Autodesk Fusion 360 part; units mm, degrees
(part 9 of 10)
  line L2725 (-28.0448, 8.6201) -> (-28.0163, 8.6133)
  line L2726 (-19.682, 10.0004) -> (-19.6496, 9.968)
  line L2727 (-19.6496, 9.968) -> (-19.645, 9.945)
  line L2728 (-19.645, 9.945) -> (-19.645, -4.025)
  line L2729 (-19.645, -4.025) -> (-19.6496, -4.048)
  line L2730 (-19.6496, -4.048) -> (-19.682, -4.0804)
  line L2731 (-19.682, -4.0804) -> (-19.705, -4.085)
  line L2732 (-19.705, -4.085) -> (-33.675, -4.085)
  line L2733 (-33.675, -4.085) -> (-33.698, -4.0804)
  line L2734 (-33.698, -4.0804) -> (-33.7304, -4.048)
  line L2735 (-33.7304, -4.048) -> (-33.735, -4.025)
  line L2736 (-33.735, -4.025) -> (-33.735, 9.945)
  line L2737 (-33.735, 9.945) -> (-33.7304, 9.968)
  line L2738 (-33.7304, 9.968) -> (-33.698, 10.0004)
  line L2739 (-33.698, 10.0004) -> (-33.675, 10.005)
  line L2740 (-33.675, 10.005) -> (-19.705, 10.005)
  line L2741 (-19.705, 10.005) -> (-19.682, 10.0004)
  line L2742 (-33.615, 9.885) -> (-33.615, -3.965)
  line L2743 (-33.615, -3.965) -> (-19.765, -3.965)
  line L2744 (-19.765, -3.965) -> (-19.765, 9.885)
  line L2745 (-19.765, 9.885) -> (-33.615, 9.885)
  line L2746 (27.428, 16.5404) -> (27.4604, 16.508)
  line L2747 (27.4604, 16.508) -> (27.465, 16.485)
  line L2748 (27.465, 16.485) -> (27.465, 2.515)
  line L2749 (27.465, 2.515) -> (27.4604, 2.492)
  line L2750 (27.4604, 2.492) -> (27.428, 2.4596)
  line L2751 (27.428, 2.4596) -> (27.405, 2.455)
  line L2752 (27.405, 2.455) -> (13.435, 2.455)
  line L2753 (13.435, 2.455) -> (13.412, 2.4596)
  line L2754 (13.412, 2.4596) -> (13.3796, 2.492)
  line L2755 (13.3796, 2.492) -> (13.375, 2.515)
  line L2756 (13.375, 2.515) -> (13.375, 16.485)
  line L2757 (13.375, 16.485) -> (13.3796, 16.508)
  line L2758 (13.3796, 16.508) -> (13.412, 16.5404)
  line L2759 (13.412, 16.5404) -> (13.435, 16.545)
  line L2760 (13.435, 16.545) -> (27.405, 16.545)
  line L2761 (27.405, 16.545) -> (27.428, 16.5404)
  line L2762 (13.495, 16.425) -> (13.495, 2.575)
  line L2763 (13.495, 2.575) -> (27.345, 2.575)
  line L2764 (27.345, 2.575) -> (27.345, 16.425)
  line L2765 (27.345, 16.425) -> (13.495, 16.425)
  line L2766 (-19.682, 25.0904) -> (-19.6496, 25.058)
  line L2767 (-19.6496, 25.058) -> (-19.645, 25.035)
  line L2768 (-19.645, 25.035) -> (-19.645, 11.065)
  line L2769 (-19.645, 11.065) -> (-19.6496, 11.042)
  line L2770 (-19.6496, 11.042) -> (-19.682, 11.0096)
  line L2771 (-19.682, 11.0096) -> (-19.705, 11.005)
  line L2772 (-19.705, 11.005) -> (-33.675, 11.005)
  line L2773 (-33.675, 11.005) -> (-33.698, 11.0096)
  line L2774 (-33.698, 11.0096) -> (-33.7304, 11.042)
  line L2775 (-33.7304, 11.042) -> (-33.735, 11.065)
  line L2776 (-33.735, 11.065) -> (-33.735, 25.035)
  line L2777 (-33.735, 25.035) -> (-33.7304, 25.058)
  line L2778 (-33.7304, 25.058) -> (-33.698, 25.0904)
  line L2779 (-33.698, 25.0904) -> (-33.675, 25.095)
  line L2780 (-33.675, 25.095) -> (-19.705, 25.095)
  line L2781 (-19.705, 25.095) -> (-19.682, 25.0904)
  line L2782 (-33.615, 24.975) -> (-33.615, 11.125)
  line L2783 (-33.615, 11.125) -> (-19.765, 11.125)
  line L2784 (-19.765, 11.125) -> (-19.765, 24.975)
  line L2785 (-19.765, 24.975) -> (-33.615, 24.975)
  line L2786 (19.0465, 17.9935) -> (19.0484, 17.9936)
  line L2787 (19.0484, 17.9936) -> (19.051, 17.993)
  line L2788 (19.051, 17.993) -> (19.0537, 17.9927)
  line L2789 (19.0537, 17.9927) -> (19.0555, 17.992)
  line L2790 (19.0555, 17.992) -> (19.0628, 17.9903)
  line L2791 (19.0628, 17.9903) -> (19.2056, 17.9427)
  line L2792 (19.2056, 17.9427) -> (19.219, 17.9367)
  line L2793 (19.219, 17.9367) -> (19.2412, 17.9175)
  line L2794 (19.2412, 17.9175) -> (19.2542, 17.8914)
  line L2795 (19.2542, 17.8914) -> (19.2563, 17.8622)
  line L2796 (19.2563, 17.8622) -> (19.2471, 17.8344)
  line L2797 (19.2471, 17.8344) -> (19.2279, 17.8123)
  line L2798 (19.2279, 17.8123) -> (19.2017, 17.7992)
  line L2799 (19.2017, 17.7992) -> (19.1725, 17.7972)
  line L2800 (19.1725, 17.7972) -> (19.1582, 17.8004)
  line L2801 (19.1582, 17.8004) -> (19.0269, 17.8442)
  line L2802 (19.0269, 17.8442) -> (18.8187, 17.8442)
  line L2803 (18.8187, 17.8442) -> (18.7501, 17.8099)
  line L2804 (18.7501, 17.8099) -> (18.7197, 17.7795)
  line L2805 (18.7197, 17.7795) -> (18.6855, 17.711)
  line L2806 (18.6855, 17.711) -> (18.6855, 17.6512)
  line L2807 (18.6855, 17.6512) -> (18.7197, 17.5827)
  line L2808 (18.7197, 17.5827) -> (18.7501, 17.5522)
  line L2809 (18.7501, 17.5522) -> (18.8271, 17.5138)
  line L2810 (18.8271, 17.5138) -> (19.0096, 17.4681)
  line L2811 (19.0096, 17.4681) -> (19.0107, 17.4677)
  line L2812 (19.0107, 17.4677) -> (19.0112, 17.4677)
  line L2813 (19.0112, 17.4677) -> (19.0173, 17.4654)
  line L2814 (19.0173, 17.4654) -> (19.0235, 17.4632)
  line L2815 (19.0235, 17.4632) -> (19.0239, 17.4629)
  line L2816 (19.0239, 17.4629) -> (19.025, 17.4625)
  line L2817 (19.025, 17.4625) -> (19.1202, 17.4148)
  line L2818 (19.1202, 17.4148) -> (19.1265, 17.4109)
  line L2819 (19.1265, 17.4109) -> (19.1283, 17.4101)
  line L2820 (19.1283, 17.4101) -> (19.1304, 17.4084)
  line L2821 (19.1304, 17.4084) -> (19.1327, 17.407)
  line L2822 (19.1327, 17.407) -> (19.1339, 17.4055)
  line L2823 (19.1339, 17.4055) -> (19.1397, 17.4008)
  line L2824 (19.1397, 17.4008) -> (19.1873, 17.3532)
  line L2825 (19.1873, 17.3532) -> (19.192, 17.3474)
  line L2826 (19.192, 17.3474) -> (19.1935, 17.3461)
  line L2827 (19.1935, 17.3461) -> (19.195, 17.3439)
  line L2828 (19.195, 17.3439) -> (19.1966, 17.3418)
  line L2829 (19.1966, 17.3418) -> (19.1974, 17.34)
  line L2830 (19.1974, 17.34) -> (19.2014, 17.3337)
  line L2831 (19.2014, 17.3337) -> (19.249, 17.2384)
  line L2832 (19.249, 17.2384) -> (19.2542, 17.2247)
  line L2833 (19.2542, 17.2247) -> (19.2544, 17.222)
  line L2834 (19.2544, 17.222) -> (19.2555, 17.2195)
  line L2835 (19.2555, 17.2195) -> (19.2569, 17.2049)
  line L2836 (19.2569, 17.2049) -> (19.2569, 17.1097)
  line L2837 (19.2569, 17.1097) -> (19.2555, 17.095)
  line L2838 (19.2555, 17.095) -> (19.2544, 17.0925)
  line L2839 (19.2544, 17.0925) -> (19.2542, 17.0898)
  line L2840 (19.2542, 17.0898) -> (19.249, 17.0761)
  line L2841 (19.249, 17.0761) -> (19.2014, 16.9809)
  line L2842 (19.2014, 16.9809) -> (19.1974, 16.9746)
  line L2843 (19.1974, 16.9746) -> (19.1966, 16.9728)
  line L2844 (19.1966, 16.9728) -> (19.195, 16.9707)
  line L2845 (19.195, 16.9707) -> (19.1935, 16.9684)
  line L2846 (19.1935, 16.9684) -> (19.192, 16.9671)
  line L2847 (19.192, 16.9671) -> (19.1873, 16.9614)
  line L2848 (19.1873, 16.9614) -> (19.1397, 16.9138)
  line L2849 (19.1397, 16.9138) -> (19.134, 16.909)
  line L2850 (19.134, 16.909) -> (19.1327, 16.9075)
  line L2851 (19.1327, 16.9075) -> (19.1304, 16.9061)
  line L2852 (19.1304, 16.9061) -> (19.1283, 16.9044)
  line L2853 (19.1283, 16.9044) -> (19.1265, 16.9037)
  line L2854 (19.1265, 16.9037) -> (19.1202, 16.8997)
  line L2855 (19.1202, 16.8997) -> (19.025, 16.8521)
  line L2856 (19.025, 16.8521) -> (19.0112, 16.8468)
  line L2857 (19.0112, 16.8468) -> (19.0085, 16.8467)
  line L2858 (19.0085, 16.8467) -> (19.0061, 16.8456)
  line L2859 (19.0061, 16.8456) -> (18.9914, 16.8442)
  line L2860 (18.9914, 16.8442) -> (18.7533, 16.8442)
  line L2861 (18.7533, 16.8442) -> (18.7459, 16.8449)
  line L2862 (18.7459, 16.8449) -> (18.744, 16.8448)
  line L2863 (18.744, 16.8448) -> (18.7414, 16.8454)
  line L2864 (18.7414, 16.8454) -> (18.7387, 16.8456)
  line L2865 (18.7387, 16.8456) -> (18.7369, 16.8464)
  line L2866 (18.7369, 16.8464) -> (18.7296, 16.848)
  line L2867 (18.7296, 16.848) -> (18.5868, 16.8956)
  line L2868 (18.5868, 16.8956) -> (18.5733, 16.9016)
  line L2869 (18.5733, 16.9016) -> (18.5512, 16.9208)
  line L2870 (18.5512, 16.9208) -> (18.5381, 16.947)
  line L2871 (18.5381, 16.947) -> (18.5361, 16.9762)
  line L2872 (18.5361, 16.9762) -> (18.5453, 17.0039)
  line L2873 (18.5453, 17.0039) -> (18.5645, 17.0261)
  line L2874 (18.5645, 17.0261) -> (18.5907, 17.0391)
  line L2875 (18.5907, 17.0391) -> (18.6199, 17.0412)
  line L2876 (18.6199, 17.0412) -> (18.6342, 17.038)
  line L2877 (18.6342, 17.038) -> (18.7655, 16.9942)
  line L2878 (18.7655, 16.9942) -> (18.9737, 16.9942)
  line L2879 (18.9737, 16.9942) -> (19.0422, 17.0284)
  line L2880 (19.0422, 17.0284) -> (19.0726, 17.0588)
  line L2881 (19.0726, 17.0588) -> (19.1069, 17.1274)
  line L2882 (19.1069, 17.1274) -> (19.1069, 17.1872)
  line L2883 (19.1069, 17.1872) -> (19.0726, 17.2557)
  line L2884 (19.0726, 17.2557) -> (19.0422, 17.2861)
  line L2885 (19.0422, 17.2861) -> (18.9653, 17.3246)
  line L2886 (18.9653, 17.3246) -> (18.7828, 17.3702)
  line L2887 (18.7828, 17.3702) -> (18.7817, 17.3706)
  line L2888 (18.7817, 17.3706) -> (18.7811, 17.3707)
  line L2889 (18.7811, 17.3707) -> (18.7751, 17.373)
  line L2890 (18.7751, 17.373) -> (18.7689, 17.3752)
  line L2891 (18.7689, 17.3752) -> (18.7685, 17.3755)
  line L2892 (18.7685, 17.3755) -> (18.7674, 17.3759)
  line L2893 (18.7674, 17.3759) -> (18.6722, 17.4235)
  line L2894 (18.6722, 17.4235) -> (18.6659, 17.4275)
  line L2895 (18.6659, 17.4275) -> (18.664, 17.4282)
  line L2896 (18.664, 17.4282) -> (18.662, 17.4299)
  line L2897 (18.662, 17.4299) -> (18.6597, 17.4314)
  line L2898 (18.6597, 17.4314) -> (18.6584, 17.4329)
  line L2899 (18.6584, 17.4329) -> (18.6527, 17.4376)
  line L2900 (18.6527, 17.4376) -> (18.6051, 17.4852)
  line L2901 (18.6051, 17.4852) -> (18.6003, 17.4909)
  line L2902 (18.6003, 17.4909) -> (18.5988, 17.4922)
  line L2903 (18.5988, 17.4922) -> (18.5974, 17.4945)
  line L2904 (18.5974, 17.4945) -> (18.5957, 17.4966)
  line L2905 (18.5957, 17.4966) -> (18.595, 17.4984)
  line L2906 (18.595, 17.4984) -> (18.591, 17.5047)
  line L2907 (18.591, 17.5047) -> (18.5434, 17.5999)
  line L2908 (18.5434, 17.5999) -> (18.5381, 17.6137)
  line L2909 (18.5381, 17.6137) -> (18.5379, 17.6163)
  line L2910 (18.5379, 17.6163) -> (18.5369, 17.6188)
  line L2911 (18.5369, 17.6188) -> (18.5355, 17.6335)
  line L2912 (18.5355, 17.6335) -> (18.5355, 17.7287)
  line L2913 (18.5355, 17.7287) -> (18.5369, 17.7433)
  line L2914 (18.5369, 17.7433) -> (18.5379, 17.7458)
  line L2915 (18.5379, 17.7458) -> (18.5381, 17.7485)
  line L2916 (18.5381, 17.7485) -> (18.5434, 17.7622)
  line L2917 (18.5434, 17.7622) -> (18.591, 17.8575)
  line L2918 (18.591, 17.8575) -> (18.595, 17.8638)
  line L2919 (18.595, 17.8638) -> (18.5957, 17.8656)
  line L2920 (18.5957, 17.8656) -> (18.5974, 17.8677)
  line L2921 (18.5974, 17.8677) -> (18.5988, 17.8699)
  line L2922 (18.5988, 17.8699) -> (18.6003, 17.8712)
  line L2923 (18.6003, 17.8712) -> (18.6051, 17.877)
  line L2924 (18.6051, 17.877) -> (18.6527, 17.9246)
  line L2925 (18.6527, 17.9246) -> (18.6584, 17.9293)
  line L2926 (18.6584, 17.9293) -> (18.6597, 17.9308)
  line L2927 (18.6597, 17.9308) -> (18.662, 17.9322)
  line L2928 (18.662, 17.9322) -> (18.664, 17.9339)
  line L2929 (18.664, 17.9339) -> (18.6659, 17.9347)
  line L2930 (18.6659, 17.9347) -> (18.6722, 17.9386)
  line L2931 (18.6722, 17.9386) -> (18.7674, 17.9863)
  line L2932 (18.7674, 17.9863) -> (18.7811, 17.9915)
  line L2933 (18.7811, 17.9915) -> (18.7838, 17.9917)
  line L2934 (18.7838, 17.9917) -> (18.7863, 17.9927)
  line L2935 (18.7863, 17.9927) -> (18.801, 17.9942)
  line L2936 (18.801, 17.9942) -> (19.039, 17.9942)
  line L2937 (19.039, 17.9942) -> (19.0465, 17.9935)
  line L2938 (20.9986, 17.9927) -> (21.0061, 17.9927)
  line L2939 (21.0061, 17.9927) -> (21.0128, 17.9899)
  line L2940 (21.0128, 17.9899) -> (21.0201, 17.9885)
  line L2941 (21.0201, 17.9885) -> (21.0262, 17.9844)
  line L2942 (21.0262, 17.9844) -> (21.0331, 17.9815)
  line L2943 (21.0331, 17.9815) -> (21.0383, 17.9763)
  line L2944 (21.0383, 17.9763) -> (21.0444, 17.9723)
  line L2945 (21.0444, 17.9723) -> (21.0485, 17.9661)
  line L2946 (21.0485, 17.9661) -> (21.0538, 17.9608)
  line L2947 (21.0538, 17.9608) -> (21.0566, 17.9541)
  line L2948 (21.0566, 17.9541) -> (21.0607, 17.948)
  line L2949 (21.0607, 17.948) -> (21.0621, 17.9407)
  line L2950 (21.0621, 17.9407) -> (21.065, 17.9338)
  line L2951 (21.065, 17.9338) -> (21.0664, 17.9193)
  line L2952 (26.0664, 17.9193) -> (26.0664, 17.9193)
  line L2953 (26.0664, 17.9193) -> (26.0664, 17.9192)
  line L2954 (26.0664, 17.9192) -> (26.0664, 17.9192)
  line L2955 (21.0664, 17.9192) -> (21.0664, 16.9942)
  line L2956 (21.0664, 16.9942) -> (21.2771, 16.9942)
  line L2957 (21.2771, 16.9942) -> (21.2918, 16.9927)
  line L2958 (21.2918, 16.9927) -> (21.3188, 16.9815)
  line L2959 (21.3188, 16.9815) -> (21.3395, 16.9608)
  line L2960 (21.3395, 16.9608) -> (21.3507, 16.9338)
  line L2961 (21.3507, 16.9338) -> (21.3507, 16.9045)
  line L2962 (21.3507, 16.9045) -> (21.3395, 16.8775)
  line L2963 (21.3395, 16.8775) -> (21.3188, 16.8568)
  line L2964 (21.3188, 16.8568) -> (21.2918, 16.8456)
  line L2965 (21.2918, 16.8456) -> (21.2771, 16.8442)
  line L2966 (21.2771, 16.8442) -> (20.7057, 16.8442)
  line L2967 (20.7057, 16.8442) -> (20.6911, 16.8456)
  line L2968 (20.6911, 16.8456) -> (20.664, 16.8568)
  line L2969 (20.664, 16.8568) -> (20.6434, 16.8775)
  line L2970 (20.6434, 16.8775) -> (20.6322, 16.9045)
  line L2971 (20.6322, 16.9045) -> (20.6322, 16.9338)
  line L2972 (20.6322, 16.9338) -> (20.6434, 16.9608)
  line L2973 (20.6434, 16.9608) -> (20.664, 16.9815)
  line L2974 (20.664, 16.9815) -> (20.6911, 16.9927)
  line L2975 (20.6911, 16.9927) -> (20.7057, 16.9942)
  line L2976 (20.7057, 16.9942) -> (20.9164, 16.9942)
  line L2977 (20.9164, 16.9942) -> (20.9164, 17.6905)
  line L2978 (20.9164, 17.6905) -> (20.854, 17.6281)
  line L2979 (20.854, 17.6281) -> (20.8482, 17.6233)
  line L2980 (20.8482, 17.6233) -> (20.8469, 17.6218)
  line L2981 (20.8469, 17.6218) -> (20.8447, 17.6204)
  line L2982 (20.8447, 17.6204) -> (20.8426, 17.6187)
  line L2983 (20.8426, 17.6187) -> (20.8408, 17.618)
  line L2984 (20.8408, 17.618) -> (20.8345, 17.614)
  line L2985 (20.8345, 17.614) -> (20.7393, 17.5664)
  line L2986 (20.7393, 17.5664) -> (20.7255, 17.5611)
  line L2987 (20.7255, 17.5611) -> (20.6963, 17.5591)
  line L2988 (20.6963, 17.5591) -> (20.6686, 17.5683)
  line L2989 (20.6686, 17.5683) -> (20.6465, 17.5875)
  line L2990 (20.6465, 17.5875) -> (20.6334, 17.6137)
  line L2991 (20.6334, 17.6137) -> (20.6313, 17.6428)
  line L2992 (20.6313, 17.6428) -> (20.6406, 17.6706)
  line L2993 (20.6406, 17.6706) -> (20.6597, 17.6927)
  line L2994 (20.6597, 17.6927) -> (20.6722, 17.7005)
  line L2995 (20.6722, 17.7005) -> (20.7565, 17.7427)
  line L2996 (20.7565, 17.7427) -> (20.8379, 17.8241)
  line L2997 (20.8379, 17.8241) -> (20.929, 17.9608)
  line L2998 (25.929, 17.9608) -> (25.9291, 17.9608)
  line L2999 (25.9291, 17.9608) -> (25.9291, 17.9608)
  line L3000 (25.9291, 17.9608) -> (25.9291, 17.9609)
  line L3001 (20.9291, 17.9609) -> (20.9383, 17.9722)
  line L3002 (20.9383, 17.9722) -> (20.9445, 17.9763)
  line L3003 (20.9445, 17.9763) -> (20.9498, 17.9815)
  line L3004 (20.9498, 17.9815) -> (20.9565, 17.9844)
  line L3005 (20.9565, 17.9844) -> (20.9627, 17.9884)
  line L3006 (20.9627, 17.9884) -> (20.9699, 17.9899)
  line L3007 (20.9699, 17.9899) -> (20.9768, 17.9927)
  line L3008 (20.9768, 17.9927) -> (20.9841, 17.9927)
  line L3009 (20.9841, 17.9927) -> (20.9913, 17.9942)
  line L3010 (20.9913, 17.9942) -> (20.9986, 17.9927)
  line L3011 (22.0061, 17.9927) -> (22.0085, 17.9917)
  line L3012 (22.0085, 17.9917) -> (22.0112, 17.9915)
  line L3013 (22.0112, 17.9915) -> (22.025, 17.9863)
  line L3014 (22.025, 17.9863) -> (22.1202, 17.9386)
  line L3015 (22.1202, 17.9386) -> (22.1265, 17.9347)
  line L3016 (22.1265, 17.9347) -> (22.1283, 17.9339)
  line L3017 (22.1283, 17.9339) -> (22.1304, 17.9322)
  line L3018 (22.1304, 17.9322) -> (22.1327, 17.9308)
  line L3019 (22.1327, 17.9308) -> (22.1339, 17.9293)
  line L3020 (22.1339, 17.9293) -> (22.1397, 17.9246)
  line L3021 (22.1397, 17.9246) -> (22.1873, 17.877)
  line L3022 (22.1873, 17.877) -> (22.192, 17.8712)
  line L3023 (22.192, 17.8712) -> (22.1935, 17.8699)
  line L3024 (22.1935, 17.8699) -> (22.195, 17.8677)
  line L3025 (22.195, 17.8677) -> (22.1966, 17.8656)
  line L3026 (22.1966, 17.8656) -> (22.1974, 17.8638)
  line L3027 (22.1974, 17.8638) -> (22.2014, 17.8575)
  line L3028 (22.2014, 17.8575) -> (22.249, 17.7622)
  line L3029 (22.249, 17.7622) -> (22.2494, 17.7612)
  line L3030 (22.2494, 17.7612) -> (22.2497, 17.7607)
  line L3031 (22.2497, 17.7607) -> (22.2519, 17.7546)
  line L3032 (22.2519, 17.7546) -> (22.2542, 17.7485)
  line L3033 (22.2542, 17.7485) -> (22.2543, 17.748)
  line L3034 (22.2543, 17.748) -> (22.2547, 17.7469)
  line L3035 (22.2547, 17.7469) -> (22.3023, 17.5564)
  line L3036 (22.3023, 17.5564) -> (22.3027, 17.5539)
  line L3037 (22.3027, 17.5539) -> (22.3031, 17.5529)
  line L3038 (22.3031, 17.5529) -> (22.3036, 17.5473)
  line L3039 (22.3036, 17.5473) -> (22.3044, 17.5419)
  line L3040 (22.3044, 17.5419) -> (22.3043, 17.5408)
  line L3041 (22.3043, 17.5408) -> (22.3045, 17.5382)
  line L3042 (22.3045, 17.5382) -> (22.3045, 17.3001)
  line L3043 (22.3045, 17.3001) -> (22.3043, 17.2976)
  line L3044 (22.3043, 17.2976) -> (22.3044, 17.2965)
  line L3045 (22.3044, 17.2965) -> (22.3036, 17.291)
  line L3046 (22.3036, 17.291) -> (22.3031, 17.2855)
  line L3047 (22.3031, 17.2855) -> (22.3027, 17.2845)
  line L3048 (22.3027, 17.2845) -> (22.3023, 17.2819)
  line L3049 (22.3023, 17.2819) -> (22.2547, 17.0915)
  line L3050 (22.2547, 17.0915) -> (22.2543, 17.0904)
  line L3051 (22.2543, 17.0904) -> (22.2542, 17.0898)
  line L3052 (22.2542, 17.0898) -> (22.2519, 17.0838)
  line L3053 (22.2519, 17.0838) -> (22.2497, 17.0776)
  line L3054 (22.2497, 17.0776) -> (22.2494, 17.0772)
  line L3055 (22.2494, 17.0772) -> (22.249, 17.0761)
  line L3056 (22.249, 17.0761) -> (22.2014, 16.9809)
  line L3057 (22.2014, 16.9809) -> (22.1974, 16.9746)
  line L3058 (22.1974, 16.9746) -> (22.1966, 16.9728)
  line L3059 (22.1966, 16.9728) -> (22.195, 16.9707)
  line L3060 (22.195, 16.9707) -> (22.1935, 16.9684)
  line L3061 (22.1935, 16.9684) -> (22.192, 16.9671)
  line L3062 (22.192, 16.9671) -> (22.1873, 16.9614)
  line L3063 (22.1873, 16.9614) -> (22.1397, 16.9138)
  line L3064 (22.1397, 16.9138) -> (22.134, 16.909)
  line L3065 (22.134, 16.909) -> (22.1327, 16.9075)
  line L3066 (22.1327, 16.9075) -> (22.1304, 16.9061)
  line L3067 (22.1304, 16.9061) -> (22.1283, 16.9044)
  line L3068 (22.1283, 16.9044) -> (22.1265, 16.9037)
  line L3069 (22.1265, 16.9037) -> (22.1202, 16.8997)
  line L3070 (22.1202, 16.8997) -> (22.025, 16.8521)
  line L3071 (22.025, 16.8521) -> (22.0112, 16.8468)
  line L3072 (22.0112, 16.8468) -> (22.0085, 16.8467)
  line L3073 (22.0085, 16.8467) -> (22.0061, 16.8456)
  line L3074 (22.0061, 16.8456) -> (21.9914, 16.8442)
  line L3075 (21.9914, 16.8442) -> (21.8962, 16.8442)
  line L3076 (21.8962, 16.8442) -> (21.8816, 16.8456)
  line L3077 (21.8816, 16.8456) -> (21.8791, 16.8467)
  line L3078 (21.8791, 16.8467) -> (21.8764, 16.8468)
  line L3079 (21.8764, 16.8468) -> (21.8626, 16.8521)
  line L3080 (21.8626, 16.8521) -> (21.7674, 16.8997)
  line L3081 (21.7674, 16.8997) -> (21.7611, 16.9037)
  line L3082 (21.7611, 16.9037) -> (21.7593, 16.9044)
  line L3083 (21.7593, 16.9044) -> (21.7572, 16.9061)
  line L3084 (21.7572, 16.9061) -> (21.755, 16.9075)
  line L3085 (21.755, 16.9075) -> (21.7537, 16.909)
  line L3086 (21.7537, 16.909) -> (21.7479, 16.9138)
  line L3087 (21.7479, 16.9138) -> (21.7003, 16.9614)
  line L3088 (21.7003, 16.9614) -> (21.6956, 16.9671)
  line L3089 (21.6956, 16.9671) -> (21.6941, 16.9684)
  line L3090 (21.6941, 16.9684) -> (21.6927, 16.9707)
  line L3091 (21.6927, 16.9707) -> (21.691, 16.9728)
  line L3092 (21.691, 16.9728) -> (21.6902, 16.9746)
  line L3093 (21.6902, 16.9746) -> (21.6863, 16.9809)
  line L3094 (21.6863, 16.9809) -> (21.6386, 17.0761)
  line L3095 (21.6386, 17.0761) -> (21.6382, 17.0772)
  line L3096 (21.6382, 17.0772) -> (21.6379, 17.0776)
  line L3097 (21.6379, 17.0776) -> (21.6357, 17.0838)
  line L3098 (21.6357, 17.0838) -> (21.6334, 17.0898)
  line L3099 (21.6334, 17.0898) -> (21.6333, 17.0904)
  line L3100 (21.6333, 17.0904) -> (21.633, 17.0915)
  line L3101 (21.633, 17.0915) -> (21.5853, 17.2819)
  line L3102 (21.5853, 17.2819) -> (21.585, 17.2845)
  line L3103 (21.585, 17.2845) -> (21.5845, 17.2855)
  line L3104 (21.5845, 17.2855) -> (21.584, 17.291)
  line L3105 (21.584, 17.291) -> (21.5832, 17.2965)
  line L3106 (21.5832, 17.2965) -> (21.5833, 17.2976)
  line L3107 (21.5833, 17.2976) -> (21.5831, 17.3001)
  line L3108 (21.5831, 17.3001) -> (21.5831, 17.5382)
  line L3109 (21.5831, 17.5382) -> (21.5833, 17.5408)
  line L3110 (21.5833, 17.5408) -> (21.5832, 17.5419)
  line L3111 (21.5832, 17.5419) -> (21.584, 17.5473)
  line L3112 (21.584, 17.5473) -> (21.5845, 17.5529)
  line L3113 (21.5845, 17.5529) -> (21.585, 17.5539)
  line L3114 (21.585, 17.5539) -> (21.5853, 17.5564)
  line L3115 (21.5853, 17.5564) -> (21.633, 17.7469)
  line L3116 (21.633, 17.7469) -> (21.6333, 17.748)
  line L3117 (21.6333, 17.748) -> (21.6334, 17.7485)
  line L3118 (21.6334, 17.7485) -> (21.6357, 17.7546)
  line L3119 (21.6357, 17.7546) -> (21.6379, 17.7607)
  line L3120 (21.6379, 17.7607) -> (21.6382, 17.7612)
  line L3121 (21.6382, 17.7612) -> (21.6386, 17.7622)
  line L3122 (21.6386, 17.7622) -> (21.6863, 17.8575)
  line L3123 (21.6863, 17.8575) -> (21.6902, 17.8638)
  line L3124 (21.6902, 17.8638) -> (21.691, 17.8656)
  line L3125 (21.691, 17.8656) -> (21.6927, 17.8677)
  line L3126 (21.6927, 17.8677) -> (21.6941, 17.8699)
  line L3127 (21.6941, 17.8699) -> (21.6956, 17.8712)
  line L3128 (21.6956, 17.8712) -> (21.7003, 17.877)
  line L3129 (21.7003, 17.877) -> (21.7479, 17.9246)
  line L3130 (21.7479, 17.9246) -> (21.7537, 17.9293)
  line L3131 (21.7537, 17.9293) -> (21.755, 17.9308)
  line L3132 (21.755, 17.9308) -> (21.7572, 17.9322)
  line L3133 (21.7572, 17.9322) -> (21.7593, 17.9339)
  line L3134 (21.7593, 17.9339) -> (21.7611, 17.9347)
  line L3135 (21.7611, 17.9347) -> (21.7674, 17.9386)
  line L3136 (21.7674, 17.9386) -> (21.8626, 17.9863)
  line L3137 (21.8626, 17.9863) -> (21.8764, 17.9915)
  line L3138 (21.8764, 17.9915) -> (21.8791, 17.9917)
  line L3139 (21.8791, 17.9917) -> (21.8816, 17.9927)
  line L3140 (21.8816, 17.9927) -> (21.8962, 17.9942)
  line L3141 (21.8962, 17.9942) -> (21.9914, 17.9942)
  line L3142 (21.9914, 17.9942) -> (22.0061, 17.9927)
  line L3143 (21.8454, 17.8099) -> (21.815, 17.7795)
  line L3144 (21.815, 17.7795) -> (21.7765, 17.7025)
  line L3145 (21.7765, 17.7025) -> (21.7331, 17.529)
  line L3146 (21.7331, 17.529) -> (21.7331, 17.3094)
  line L3147 (21.7331, 17.3094) -> (21.7765, 17.1358)
  line L3148 (21.7765, 17.1358) -> (21.815, 17.0588)
  line L3149 (21.815, 17.0588) -> (21.8454, 17.0284)
  line L3150 (21.8454, 17.0284) -> (21.9139, 16.9942)
  line L3151 (21.9139, 16.9942) -> (21.9737, 16.9942)
  line L3152 (21.9737, 16.9942) -> (22.0422, 17.0284)
  line L3153 (22.0422, 17.0284) -> (22.0726, 17.0588)
  line L3154 (22.0726, 17.0588) -> (22.1111, 17.1358)
  line L3155 (22.1111, 17.1358) -> (22.1545, 17.3094)
  line L3156 (22.1545, 17.3094) -> (22.1545, 17.529)
  line L3157 (22.1545, 17.529) -> (22.1111, 17.7025)
  line L3158 (22.1111, 17.7025) -> (22.0726, 17.7795)
  line L3159 (22.0726, 17.7795) -> (22.0422, 17.8099)
  line L3160 (22.0422, 17.8099) -> (21.9737, 17.8442)
  line L3161 (21.9737, 17.8442) -> (21.9139, 17.8442)
  line L3162 (21.9139, 17.8442) -> (21.8454, 17.8099)
  line L3163 (20.4037, 17.9874) -> (20.4274, 17.9702)
  line L3164 (20.4274, 17.9702) -> (20.4427, 17.9453)
  line L3165 (20.4427, 17.9453) -> (20.4473, 17.9164)
  line L3166 (20.4473, 17.9164) -> (20.4453, 17.9018)
  line L3167 (20.4453, 17.9018) -> (20.2072, 16.9018)
  line L3168 (20.2072, 16.9018) -> (20.2055, 16.8968)
  line L3169 (20.2055, 16.8968) -> (20.2053, 16.895)
  line L3170 (20.2053, 16.895) -> (20.2043, 16.8934)
  line L3171 (20.2043, 16.8934) -> (20.2025, 16.8879)
  line L3172 (20.2025, 16.8879) -> (20.1961, 16.8791)
  line L3173 (20.1961, 16.8791) -> (20.1906, 16.8697)
  line L3174 (20.1906, 16.8697) -> (20.1876, 16.8673)
  line L3175 (20.1876, 16.8673) -> (20.1853, 16.8642)
  line L3176 (20.1853, 16.8642) -> (20.176, 16.8585)
  line L3177 (20.176, 16.8585) -> (20.1674, 16.8519)
  line L3178 (20.1674, 16.8519) -> (20.1637, 16.8509)
  line L3179 (20.1637, 16.8509) -> (20.1604, 16.8489)
  line L3180 (20.1604, 16.8489) -> (20.1496, 16.8471)
  line L3181 (20.1496, 16.8471) -> (20.1391, 16.8443)
  line L3182 (20.1391, 16.8443) -> (20.1353, 16.8448)
  line L3183 (20.1353, 16.8448) -> (20.1315, 16.8442)
  line L3184 (20.1315, 16.8442) -> (20.1209, 16.8468)
  line L3185 (20.1209, 16.8468) -> (20.1101, 16.8482)
  line L3186 (20.1101, 16.8482) -> (20.1068, 16.8501)
  line L3187 (20.1068, 16.8501) -> (20.103, 16.851)
  line L3188 (20.103, 16.851) -> (20.0942, 16.8574)
  line L3189 (20.0942, 16.8574) -> (20.0848, 16.8629)
  line L3190 (20.0848, 16.8629) -> (20.0824, 16.8659)
  line L3191 (20.0824, 16.8659) -> (20.0793, 16.8682)
  line L3192 (20.0793, 16.8682) -> (20.0736, 16.8774)
  line L3193 (20.0736, 16.8774) -> (20.067, 16.8861)
  line L3194 (20.067, 16.8861) -> (20.065, 16.8915)
  line L3195 (20.065, 16.8915) -> (20.064, 16.8931)
  line L3196 (20.064, 16.8931) -> (20.0637, 16.8949)
  line L3197 (20.0637, 16.8949) -> (20.0618, 16.8999)
  line L3198 (20.0618, 16.8999) -> (19.9438, 17.3424)
  line L3199 (19.9438, 17.3424) -> (19.8258, 16.8999)
  line L3200 (19.8258, 16.8999) -> (19.8239, 16.8949)
  line L3201 (19.8239, 16.8949) -> (19.8236, 16.8931)
  line L3202 (19.8236, 16.8931) -> (19.8227, 16.8915)
  line L3203 (19.8227, 16.8915) -> (19.8206, 16.8861)
  line L3204 (19.8206, 16.8861) -> (19.814, 16.8774)
  line L3205 (19.814, 16.8774) -> (19.8083, 16.8682)
  line L3206 (19.8083, 16.8682) -> (19.8052, 16.8659)
  line L3207 (19.8052, 16.8659) -> (19.8029, 16.8629)
  line L3208 (19.8029, 16.8629) -> (19.7934, 16.8574)
  line L3209 (19.7934, 16.8574) -> (19.7846, 16.851)
  line L3210 (19.7846, 16.851) -> (19.7809, 16.8501)
  line L3211 (19.7809, 16.8501) -> (19.7775, 16.8482)
  line L3212 (19.7775, 16.8482) -> (19.7667, 16.8468)
  line L3213 (19.7667, 16.8468) -> (19.7561, 16.8442)
  line L3214 (19.7561, 16.8442) -> (19.7523, 16.8448)
  line L3215 (19.7523, 16.8448) -> (19.7485, 16.8443)
  line L3216 (19.7485, 16.8443) -> (19.738, 16.8471)
  line L3217 (19.738, 16.8471) -> (19.7272, 16.8489)
  line L3218 (19.7272, 16.8489) -> (19.724, 16.8509)
  line L3219 (19.724, 16.8509) -> (19.7202, 16.8519)
  line L3220 (19.7202, 16.8519) -> (19.7116, 16.8585)
  line L3221 (19.7116, 16.8585) -> (19.7023, 16.8642)
  line L3222 (19.7023, 16.8642) -> (19.7001, 16.8673)
  line L3223 (19.7001, 16.8673) -> (19.697, 16.8697)
  line L3224 (19.697, 16.8697) -> (19.6915, 16.8791)
  line L3225 (19.6915, 16.8791) -> (19.6852, 16.8879)
  line L3226 (19.6852, 16.8879) -> (19.6833, 16.8934)
  line L3227 (19.6833, 16.8934) -> (19.6823, 16.895)
  line L3228 (19.6823, 16.895) -> (19.6821, 16.8968)
  line L3229 (19.6821, 16.8968) -> (19.6804, 16.9018)
  line L3230 (19.6804, 16.9018) -> (19.4423, 17.9018)
  line L3231 (19.4423, 17.9018) -> (19.4403, 17.9164)
  line L3232 (19.4403, 17.9164) -> (19.4449, 17.9453)
  line L3233 (19.4449, 17.9453) -> (19.4603, 17.9702)
  line L3234 (19.4603, 17.9702) -> (19.484, 17.9874)
  line L3235 (19.484, 17.9874) -> (19.5124, 17.9941)
  line L3236 (19.5124, 17.9941) -> (19.5413, 17.9895)
  line L3237 (19.5413, 17.9895) -> (19.5663, 17.9742)
  line L3238 (19.5663, 17.9742) -> (19.5834, 17.9505)
  line L3239 (19.5834, 17.9505) -> (19.5882, 17.9366)
  line L3240 (19.5882, 17.9366) -> (19.7574, 17.2257)
  line L3241 (19.7574, 17.2257) -> (19.8713, 17.6528)
  line L3242 (19.8713, 17.6528) -> (19.8726, 17.6562)
  line L3243 (19.8726, 17.6562) -> (19.8728, 17.6577)
  line L3244 (19.8728, 17.6577) -> (19.8738, 17.6594)
  line L3245 (19.8738, 17.6594) -> (19.8765, 17.6666)
  line L3246 (19.8765, 17.6666) -> (19.8825, 17.6744)
  line L3247 (19.8825, 17.6744) -> (19.8875, 17.683)
  line L3248 (19.8875, 17.683) -> (19.8913, 17.6859)
  line L3249 (19.8913, 17.6859) -> (19.8943, 17.6898)
  line L3250 (19.8943, 17.6898) -> (19.9029, 17.6948)
  line L3251 (19.9029, 17.6948) -> (19.9107, 17.7008)
  line L3252 (19.9107, 17.7008) -> (19.9154, 17.702)
  line L3253 (19.9154, 17.702) -> (19.9196, 17.7045)
  line L3254 (19.9196, 17.7045) -> (19.9294, 17.7058)
  line L3255 (19.9294, 17.7058) -> (19.939, 17.7083)
  line L3256 (19.939, 17.7083) -> (19.9438, 17.7077)
  line L3257 (19.9438, 17.7077) -> (19.9486, 17.7083)
  line L3258 (19.9486, 17.7083) -> (19.9582, 17.7058)
  line L3259 (19.9582, 17.7058) -> (19.968, 17.7045)
  line L3260 (19.968, 17.7045) -> (19.9722, 17.702)
  line L3261 (19.9722, 17.702) -> (19.9769, 17.7008)
  line L3262 (19.9769, 17.7008) -> (19.9848, 17.6948)
  line L3263 (19.9848, 17.6948) -> (19.9933, 17.6898)
  line L3264 (19.9933, 17.6898) -> (19.9963, 17.6859)
  line L3265 (19.9963, 17.6859) -> (20.0001, 17.683)
  line L3266 (20.0001, 17.683) -> (20.0051, 17.6744)
  line L3267 (20.0051, 17.6744) -> (20.0111, 17.6666)
  line L3268 (20.0111, 17.6666) -> (20.0138, 17.6594)
  line L3269 (20.0138, 17.6594) -> (20.0148, 17.6577)
  line L3270 (20.0148, 17.6577) -> (20.015, 17.6562)
  line L3271 (20.015, 17.6562) -> (20.0163, 17.6528)
  line L3272 (20.0163, 17.6528) -> (20.1302, 17.2257)
  line L3273 (20.1302, 17.2257) -> (20.2994, 17.9366)
  line L3274 (20.2994, 17.9366) -> (20.3042, 17.9505)
  line L3275 (20.3042, 17.9505) -> (20.3214, 17.9742)
  line L3276 (20.3214, 17.9742) -> (20.3463, 17.9895)
  line L3277 (20.3463, 17.9895) -> (20.3752, 17.9941)
  line L3278 (20.3752, 17.9941) -> (20.4037, 17.9874)
  line L3279 (-0.5862, 50.7707) -> (-0.5518, 50.7363)
  line L3280 (-0.5518, 50.7363) -> (-0.547, 50.712)
  line L3281 (-0.547, 50.712) -> (-0.547, 49.3506)
  line L3282 (-0.547, 49.3506) -> (1.7895, 49.3506)
  line L3283 (1.7895, 49.3506) -> (1.8115, 49.3462)
  line L3284 (1.8115, 49.3462) -> (2.0576, 49.3251)
  line L3285 (2.0576, 49.3251) -> (2.3192, 49.2686)
  line L3286 (2.3192, 49.2686) -> (2.5716, 49.1793)
  line L3287 (2.5716, 49.1793) -> (2.8107, 49.0587)
  line L3288 (2.8107, 49.0587) -> (3.0325, 48.9088)
  line L3289 (3.0325, 48.9088) -> (3.2334, 48.7319)
  line L3290 (3.2334, 48.7319) -> (3.4103, 48.5309)
  line L3291 (3.4103, 48.5309) -> (3.5603, 48.3092)
  line L3292 (3.5603, 48.3092) -> (3.6808, 48.0701)
  line L3293 (3.6808, 48.0701) -> (3.7701, 47.8177)
  line L3294 (3.7701, 47.8177) -> (3.8266, 47.556)
  line L3295 (3.8266, 47.556) -> (3.8475, 47.313)
  line L3296 (3.8475, 47.313) -> (3.8482, 47.3123)
  line L3297 (3.8482, 47.3123) -> (3.853, 47.288)
  line L3298 (3.853, 47.288) -> (3.853, 30.288)
  line L3299 (3.853, 30.288) -> (3.8482, 30.2637)
  line L3300 (3.8482, 30.2637) -> (3.8479, 30.2634)
  line L3301 (3.8479, 30.2634) -> (3.8319, 30.0191)
  line L3302 (3.8319, 30.0191) -> (3.7793, 29.7548)
  line L3303 (3.7793, 29.7548) -> (3.6927, 29.4997)
  line L3304 (3.6927, 29.4997) -> (3.5735, 29.258)
  line L3305 (3.5735, 29.258) -> (3.4238, 29.0339)
  line L3306 (3.4238, 29.0339) -> (3.2461, 28.8313)
  line L3307 (3.2461, 28.8313) -> (3.0435, 28.6537)
  line L3308 (3.0435, 28.6537) -> (2.8195, 28.504)
  line L3309 (2.8195, 28.504) -> (2.5778, 28.3848)
  line L3310 (2.5778, 28.3848) -> (2.3227, 28.2982)
  line L3311 (2.3227, 28.2982) -> (2.0584, 28.2456)
  line L3312 (2.0584, 28.2456) -> (1.8141, 28.2296)
  line L3313 (1.8141, 28.2296) -> (1.8138, 28.2293)
  line L3314 (1.8138, 28.2293) -> (1.7895, 28.2245)
  line L3315 (1.7895, 28.2245) -> (-12.0105, 28.2245)
  line L3316 (-12.0105, 28.2245) -> (-12.0348, 28.2293)
  line L3317 (-12.0348, 28.2293) -> (-12.0355, 28.23)
  line L3318 (-12.0355, 28.23) -> (-12.2785, 28.2509)
  line L3319 (-12.2785, 28.2509) -> (-12.5402, 28.3074)
  line L3320 (-12.5402, 28.3074) -> (-12.7926, 28.3967)
  line L3321 (-12.7926, 28.3967) -> (-13.0316, 28.5173)
  line L3322 (-13.0316, 28.5173) -> (-13.2534, 28.6673)
  line L3323 (-13.2534, 28.6673) -> (-13.4543, 28.8441)
  line L3324 (-13.4543, 28.8441) -> (-13.6312, 29.0451)
  line L3325 (-13.6312, 29.0451) -> (-13.7812, 29.2669)
  line L3326 (-13.7812, 29.2669) -> (-13.9018, 29.5059)
  line L3327 (-13.9018, 29.5059) -> (-13.9911, 29.7583)
  line L3328 (-13.9911, 29.7583) -> (-14.0476, 30.0199)
  line L3329 (-14.0476, 30.0199) -> (-14.0685, 30.263)
  line L3330 (-14.0685, 30.263) -> (-14.0692, 30.2637)
  line L3331 (-14.0692, 30.2637) -> (-14.074, 30.288)
  line L3332 (-14.074, 30.288) -> (-14.074, 47.288)
  line L3333 (-14.074, 47.288) -> (-14.0692, 47.3123)
  line L3334 (-14.0692, 47.3123) -> (-14.0685, 47.313)
  line L3335 (-14.0685, 47.313) -> (-14.0476, 47.556)
  line L3336 (-14.0476, 47.556) -> (-13.9911, 47.8177)
  line L3337 (-13.9911, 47.8177) -> (-13.9018, 48.0701)
  line L3338 (-13.9018, 48.0701) -> (-13.7813, 48.3092)
  line L3339 (-13.7813, 48.3092) -> (-13.6313, 48.5309)
  line L3340 (-13.6313, 48.5309) -> (-13.4544, 48.7319)
  line L3341 (-13.4544, 48.7319) -> (-13.2535, 48.9088)
  line L3342 (-13.2535, 48.9088) -> (-13.0317, 49.0587)
  line L3343 (-13.0317, 49.0587) -> (-12.7926, 49.1793)
  line L3344 (-12.7926, 49.1793) -> (-12.5402, 49.2686)
  line L3345 (-12.5402, 49.2686) -> (-12.2786, 49.3251)
  line L3346 (-12.2786, 49.3251) -> (-12.0325, 49.3462)
  line L3347 (-12.0325, 49.3462) -> (-12.0105, 49.3506)
  line L3348 (-12.0105, 49.3506) -> (-9.674, 49.3506)
  line L3349 (-9.674, 49.3506) -> (-9.674, 50.712)
  line L3350 (-9.674, 50.712) -> (-9.6692, 50.7363)
  line L3351 (-9.6692, 50.7363) -> (-9.6348, 50.7707)
  line L3352 (-9.6348, 50.7707) -> (-9.6105, 50.7755)
  line L3353 (-9.6105, 50.7755) -> (-0.6105, 50.7755)
  line L3354 (-0.6105, 50.7755) -> (-0.5862, 50.7707)
  line L3355 (1.7895, 49.2236) -> (-0.547, 49.2236)
  line L3356 (-0.547, 49.2236) -> (-0.547, 43.3587)
  line L3357 (-0.547, 43.3587) -> (-0.5518, 43.3344)
  line L3358 (-0.5518, 43.3344) -> (-0.5862, 43.3)
  line L3359 (-0.5862, 43.3) -> (-0.6105, 43.2952)
  line L3360 (-0.6105, 43.2952) -> (-9.6105, 43.2952)
  line L3361 (-9.6105, 43.2952) -> (-9.6348, 43.3)
  line L3362 (-9.6348, 43.3) -> (-9.6692, 43.3344)
  line L3363 (-9.6692, 43.3344) -> (-9.674, 43.3587)
  line L3364 (-9.674, 43.3587) -> (-9.674, 49.2236)
  line L3365 (-9.674, 49.2236) -> (-12.0105, 49.2236)
  line L3366 (-12.0105, 49.2236) -> (-12.0305, 49.2275)
  line L3367 (-12.0305, 49.2275) -> (-12.1357, 49.2253)
  line L3368 (-12.1357, 49.2253) -> (-12.3858, 49.1877)
  line L3369 (-12.3858, 49.1877) -> (-12.6292, 49.1187)
  line L3370 (-12.6292, 49.1187) -> (-12.8619, 49.0193)
  line L3371 (-12.8619, 49.0193) -> (-13.08, 48.8913)
  line L3372 (-13.08, 48.8913) -> (-13.2802, 48.7365)
  line L3373 (-13.2802, 48.7365) -> (-13.4591, 48.5577)
  line L3374 (-13.4591, 48.5577) -> (-13.6138, 48.3575)
  line L3375 (-13.6138, 48.3575) -> (-13.7419, 48.1393)
  line L3376 (-13.7419, 48.1393) -> (-13.8412, 47.9067)
  line L3377 (-13.8412, 47.9067) -> (-13.9102, 47.6633)
  line L3378 (-13.9102, 47.6633) -> (-13.9478, 47.4131)
  line L3379 (-13.9478, 47.4131) -> (-13.9501, 47.3038)
  line L3380 (-13.9501, 47.3038) -> (-13.947, 47.288)
  line L3381 (-13.947, 47.288) -> (-13.947, 30.288)
  line L3382 (-13.947, 30.288) -> (-13.9501, 30.2722)
  line L3383 (-13.9501, 30.2722) -> (-13.9478, 30.1628)
  line L3384 (-13.9478, 30.1628) -> (-13.9102, 29.9127)
  line L3385 (-13.9102, 29.9127) -> (-13.8412, 29.6693)
  line L3386 (-13.8412, 29.6693) -> (-13.7418, 29.4367)
  line L3387 (-13.7418, 29.4367) -> (-13.6137, 29.2185)
  line L3388 (-13.6137, 29.2185) -> (-13.459, 29.0184)
  line L3389 (-13.459, 29.0184) -> (-13.2801, 28.8395)
  line L3390 (-13.2801, 28.8395) -> (-13.08, 28.6848)
  line L3391 (-13.08, 28.6848) -> (-12.8618, 28.5567)
  line L3392 (-12.8618, 28.5567) -> (-12.6292, 28.4573)
  line L3393 (-12.6292, 28.4573) -> (-12.3858, 28.3883)
  line L3394 (-12.3858, 28.3883) -> (-12.1356, 28.3507)
  line L3395 (-12.1356, 28.3507) -> (-12.0263, 28.3483)
  line L3396 (-12.0263, 28.3483) -> (-12.0105, 28.3515)
  line L3397 (-12.0105, 28.3515) -> (1.7895, 28.3515)
  line L3398 (1.7895, 28.3515) -> (1.8071, 28.348)
  line L3399 (1.8071, 28.348) -> (1.9167, 28.348)
  line L3400 (1.9167, 28.348) -> (2.1688, 28.3812)
  line L3401 (2.1688, 28.3812) -> (2.4144, 28.447)
  line L3402 (2.4144, 28.447) -> (2.6494, 28.5443)
  line L3403 (2.6494, 28.5443) -> (2.8696, 28.6715)
  line L3404 (2.8696, 28.6715) -> (3.0714, 28.8263)
  line L3405 (3.0714, 28.8263) -> (3.2512, 29.0061)
  line L3406 (3.2512, 29.0061) -> (3.406, 29.2079)
  line L3407 (3.406, 29.2079) -> (3.5332, 29.4281)
  line L3408 (3.5332, 29.4281) -> (3.6305, 29.6631)
  line L3409 (3.6305, 29.6631) -> (3.6963, 29.9087)
  line L3410 (3.6963, 29.9087) -> (3.7295, 30.1608)
  line L3411 (3.7295, 30.1608) -> (3.7295, 30.2704)
  line L3412 (3.7295, 30.2704) -> (3.726, 30.288)
  line L3413 (3.726, 30.288) -> (3.726, 47.288)
  line L3414 (3.726, 47.288) -> (3.7291, 47.3038)
  line L3415 (3.7291, 47.3038) -> (3.7268, 47.4131)
  line L3416 (3.7268, 47.4131) -> (3.6892, 47.6633)
  line L3417 (3.6892, 47.6633) -> (3.6202, 47.9067)
  line L3418 (3.6202, 47.9067) -> (3.5209, 48.1393)
  line L3419 (3.5209, 48.1393) -> (3.3928, 48.3575)
  line L3420 (3.3928, 48.3575) -> (3.2381, 48.5577)
  line L3421 (3.2381, 48.5577) -> (3.0592, 48.7365)
  line L3422 (3.0592, 48.7365) -> (2.859, 48.8913)
  line L3423 (2.859, 48.8913) -> (2.6409, 49.0193)
  line L3424 (2.6409, 49.0193) -> (2.4082, 49.1187)
  line L3425 (2.4082, 49.1187) -> (2.1648, 49.1877)
  line L3426 (2.1648, 49.1877) -> (1.9147, 49.2253)
  line L3427 (1.9147, 49.2253) -> (1.8095, 49.2275)
  line L3428 (1.8095, 49.2275) -> (1.7895, 49.2236)
  line L3429 (-9.547, 49.2236) -> (-9.547, 43.4222)
  line L3430 (-9.547, 43.4222) -> (-0.674, 43.4222)
  line L3431 (-0.674, 43.4222) -> (-0.674, 49.2236)
  line L3432 (-0.674, 49.2236) -> (-9.547, 49.2236)
  line L3433 (-9.547, 50.6485) -> (-9.547, 49.3506)
  line L3434 (-9.547, 49.3506) -> (-0.674, 49.3506)
  line L3435 (-0.674, 49.3506) -> (-0.674, 50.6485)
  line L3436 (-0.674, 50.6485) -> (-9.547, 50.6485)
  line L3437 (-33.1806, 36.5339) -> (-33.1461, 36.4994)
  line L3438 (-33.1461, 36.4994) -> (-33.1274, 36.4544)
  line L3439 (-33.1274, 36.4544) -> (-33.125, 36.43)
  line L3440 (-33.125, 36.43) -> (-33.125, 32.725)
  line L3441 (-33.125, 32.725) -> (-21.575, 32.725)
  line L3442 (-21.575, 32.725) -> (-21.575, 36.43)
  line L3443 (-21.575, 36.43) -> (-21.5726, 36.4544)
  line L3444 (-21.5726, 36.4544) -> (-21.5539, 36.4994)
  line L3445 (-21.5539, 36.4994) -> (-21.5194, 36.5339)
  line L3446 (-21.5194, 36.5339) -> (-21.4744, 36.5526)
  line L3447 (-21.4744, 36.5526) -> (-21.4256, 36.5526)
  line L3448 (-21.4256, 36.5526) -> (-21.3806, 36.5339)
  line L3449 (-21.3806, 36.5339) -> (-21.3461, 36.4994)
  line L3450 (-21.3461, 36.4994) -> (-21.3274, 36.4544)
  line L3451 (-21.3274, 36.4544) -> (-21.325, 36.43)
  line L3452 (-21.325, 36.43) -> (-21.325, 32.6)
  line L3453 (-21.325, 32.6) -> (-21.3274, 32.5756)
  line L3454 (-21.3274, 32.5756) -> (-21.3461, 32.5306)
  line L3455 (-21.3461, 32.5306) -> (-21.3806, 32.4961)
  line L3456 (-21.3806, 32.4961) -> (-21.4256, 32.4774)
  line L3457 (-21.4256, 32.4774) -> (-21.45, 32.475)
  line L3458 (-21.45, 32.475) -> (-33.25, 32.475)
  line L3459 (-33.25, 32.475) -> (-33.2744, 32.4774)
  line L3460 (-33.2744, 32.4774) -> (-33.3194, 32.4961)
  line L3461 (-33.3194, 32.4961) -> (-33.3539, 32.5306)
  line L3462 (-33.3539, 32.5306) -> (-33.3726, 32.5756)
  line L3463 (-33.3726, 32.5756) -> (-33.375, 32.6)
  line L3464 (-33.375, 32.6) -> (-33.375, 36.43)
  line L3465 (-33.375, 36.43) -> (-33.3726, 36.4544)
  line L3466 (-33.3726, 36.4544) -> (-33.3539, 36.4994)
  line L3467 (-33.3539, 36.4994) -> (-33.3194, 36.5339)
  line L3468 (-33.3194, 36.5339) -> (-33.2744, 36.5526)
  line L3469 (-33.2744, 36.5526) -> (-33.2256, 36.5526)
  line L3470 (-33.2256, 36.5526) -> (-33.1806, 36.5339)
  line L3471 (-26.8182, 41.7301) -> (-26.471, 41.6509)
  line L3472 (-26.471, 41.6509) -> (-26.135, 41.5333)
  line L3473 (-26.135, 41.5333) -> (-25.8142, 41.3788)
  line L3474 (-25.8142, 41.3788) -> (-25.5127, 41.1894)
  line L3475 (-25.5127, 41.1894) -> (-25.2343, 40.9674)
  line L3476 (-25.2343, 40.9674) -> (-24.9826, 40.7156)
  line L3477 (-24.9826, 40.7156) -> (-24.7606, 40.4373)
  line L3478 (-24.7606, 40.4373) -> (-24.5712, 40.1358)
  line L3479 (-24.5712, 40.1358) -> (-24.4167, 39.815)
  line L3480 (-24.4167, 39.815) -> (-24.2991, 39.479)
  line L3481 (-24.2991, 39.479) -> (-24.2199, 39.1318)
  line L3482 (-24.2199, 39.1318) -> (-24.18, 38.778)
  line L3483 (-24.18, 38.778) -> (-24.18, 38.422)
  line L3484 (-24.18, 38.422) -> (-24.2199, 38.0682)
  line L3485 (-24.2199, 38.0682) -> (-24.2991, 37.721)
  line L3486 (-24.2991, 37.721) -> (-24.4167, 37.385)
  line L3487 (-24.4167, 37.385) -> (-24.5712, 37.0642)
  line L3488 (-24.5712, 37.0642) -> (-24.7606, 36.7627)
  line L3489 (-24.7606, 36.7627) -> (-24.9826, 36.4844)
  line L3490 (-24.9826, 36.4843) -> (-25.2343, 36.2326)
  line L3491 (-25.2343, 36.2326) -> (-25.5127, 36.0106)
  line L3492 (-25.5127, 36.0106) -> (-25.8142, 35.8212)
  line L3493 (-25.8142, 35.8212) -> (-26.135, 35.6667)
  line L3494 (-26.135, 35.6667) -> (-26.471, 35.5491)
  line L3495 (-26.471, 35.5491) -> (-26.8182, 35.4699)
  line L3496 (-26.8182, 35.4699) -> (-27.172, 35.43)
  line L3497 (-27.172, 35.43) -> (-27.528, 35.43)
  line L3498 (-27.528, 35.43) -> (-27.8818, 35.4699)
  line L3499 (-27.8818, 35.4699) -> (-28.229, 35.5491)
  line L3500 (-28.229, 35.5491) -> (-28.565, 35.6667)
  line L3501 (-28.565, 35.6667) -> (-28.8858, 35.8212)
  line L3502 (-28.8858, 35.8212) -> (-29.1873, 36.0106)
  line L3503 (-29.1873, 36.0106) -> (-29.4656, 36.2326)
  line L3504 (-29.4656, 36.2326) -> (-29.7174, 36.4843)
  line L3505 (-29.7174, 36.4843) -> (-29.9394, 36.7627)
  line L3506 (-29.9394, 36.7627) -> (-30.1288, 37.0642)
  line L3507 (-30.1288, 37.0642) -> (-30.2833, 37.385)
  line L3508 (-30.2833, 37.385) -> (-30.4009, 37.721)
  line L3509 (-30.4009, 37.721) -> (-30.4801, 38.0682)
  line L3510 (-30.4801, 38.0682) -> (-30.52, 38.422)
  line L3511 (-30.52, 38.422) -> (-30.52, 38.7643)
  line L3512 (-30.52, 38.7643) -> (-30.52, 38.778)
  line L3513 (-30.52, 38.778) -> (-30.4801, 39.1318)
  line L3514 (-30.4801, 39.1318) -> (-30.4009, 39.479)
  line L3515 (-30.4009, 39.479) -> (-30.2833, 39.815)
  line L3516 (-30.2833, 39.815) -> (-30.1288, 40.1358)
  line L3517 (-30.1288, 40.1358) -> (-29.9394, 40.4373)
  line L3518 (-29.9394, 40.4373) -> (-29.7174, 40.7156)
  line L3519 (-29.7174, 40.7156) -> (-29.4656, 40.9674)
  line L3520 (-29.4656, 40.9674) -> (-29.1873, 41.1894)
  line L3521 (-29.1873, 41.1894) -> (-28.8858, 41.3788)
  line L3522 (-28.8858, 41.3788) -> (-28.565, 41.5333)
  line L3523 (-28.565, 41.5333) -> (-28.229, 41.6509)
  line L3524 (-28.229, 41.6509) -> (-27.8818, 41.7301)
  line L3525 (-27.8818, 41.7301) -> (-27.528, 41.77)
  line L3526 (-27.528, 41.77) -> (-27.172, 41.77)
  line L3527 (-27.172, 41.77) -> (-26.8182, 41.7301)
  line L3528 (-29.0569, 39.495) -> (-29.0863, 39.4427)
  line L3529 (-29.0863, 39.4427) -> (-29.1834, 39.1948)
  line L3530 (-29.1834, 39.1948) -> (-29.2452, 38.9358)
  line L3531 (-29.2452, 38.9358) -> (-29.2707, 38.6707)
  line L3532 (-29.2707, 38.6707) -> (-29.2592, 38.4046)
  line L3533 (-29.2592, 38.4046) -> (-29.2111, 38.1427)
  line L3534 (-29.2111, 38.1427) -> (-29.1273, 37.89)
  line L3535 (-29.1273, 37.89) -> (-29.0093, 37.6513)
  line L3536 (-29.0093, 37.6513) -> (-28.8594, 37.4312)
  line L3537 (-28.8594, 37.4312) -> (-28.6805, 37.2339)
  line L3538 (-28.6805, 37.2339) -> (-28.4761, 37.0632)
  line L3539 (-28.4761, 37.0632) -> (-28.25, 36.9225)
  line L3540 (-28.25, 36.9225) -> (-28.0067, 36.8144)
  line L3541 (-28.0067, 36.8144) -> (-27.7507, 36.7409)
  line L3542 (-27.7507, 36.7409) -> (-27.4871, 36.7036)
  line L3543 (-27.4871, 36.7036) -> (-27.2208, 36.703)
  line L3544 (-27.2208, 36.703) -> (-26.957, 36.7393)
  line L3545 (-26.957, 36.7393) -> (-26.7007, 36.8117)
  line L3546 (-26.7007, 36.8117) -> (-26.4569, 36.9188)
  line L3547 (-26.4569, 36.9188) -> (-26.2303, 37.0586)
  line L3548 (-26.2303, 37.0586) -> (-26.0252, 37.2285)
  line L3549 (-26.0252, 37.2285) -> (-25.8455, 37.425)
  line L3550 (-25.8455, 37.425) -> (-25.6947, 37.6445)
  line L3551 (-25.6947, 37.6445) -> (-25.5757, 37.8827)
  line L3552 (-25.5757, 37.8827) -> (-25.4908, 38.1351)
  line L3553 (-25.4908, 38.1351) -> (-25.4417, 38.3968)
  line L3554 (-25.4417, 38.3968) -> (-25.4291, 38.6628)
  line L3555 (-25.4291, 38.6628) -> (-25.4535, 38.928)
  line L3556 (-25.4535, 38.928) -> (-25.5143, 39.1873)
  line L3557 (-25.5143, 39.1873) -> (-25.6104, 39.4356)
  line L3558 (-25.6104, 39.4356) -> (-25.6434, 39.495)
  line L3559 (-25.6434, 39.495) -> (-29.0569, 39.495)
  line L3560 (-27.8407, 41.4882) -> (-28.161, 41.4151)
  line L3561 (-28.161, 41.4151) -> (-28.4711, 41.3066)
  line L3562 (-28.4711, 41.3066) -> (-28.7671, 41.1641)
  line L3563 (-28.7671, 41.1641) -> (-29.0453, 40.9893)
  line L3564 (-29.0453, 40.9893) -> (-29.3021, 40.7844)
  line L3565 (-29.3021, 40.7844) -> (-29.5344, 40.5521)
  line L3566 (-29.5344, 40.5521) -> (-29.7393, 40.2953)
  line L3567 (-29.7393, 40.2953) -> (-29.9141, 40.0171)
  line L3568 (-29.9141, 40.0171) -> (-30.0451, 39.745)
  line L3569 (-30.0451, 39.745) -> (-24.6549, 39.745)
  line L3570 (-24.6549, 39.745) -> (-24.7859, 40.0171)
  line L3571 (-24.7859, 40.0171) -> (-24.9607, 40.2953)
  line L3572 (-24.9607, 40.2953) -> (-25.1656, 40.5521)
  line L3573 (-25.1656, 40.5521) -> (-25.3979, 40.7844)
  line L3574 (-25.3979, 40.7844) -> (-25.6547, 40.9893)
  line L3575 (-25.6547, 40.9893) -> (-25.9329, 41.1641)
  line L3576 (-25.9329, 41.1641) -> (-26.2289, 41.3066)
  line L3577 (-26.2289, 41.3066) -> (-26.539, 41.4151)
  line L3578 (-26.539, 41.4151) -> (-26.8593, 41.4882)
  line L3579 (-26.8593, 41.4882) -> (-27.1857, 41.525)
  line L3580 (-27.1857, 41.525) -> (-27.5143, 41.525)
  line L3581 (-27.5143, 41.525) -> (-27.8407, 41.4882)
  line L3582 (-30.275, 38.4357) -> (-30.2382, 38.1093)
  line L3583 (-30.2382, 38.1093) -> (-30.1651, 37.789)
  line L3584 (-30.1651, 37.789) -> (-30.0566, 37.4789)
  line L3585 (-30.0566, 37.4789) -> (-29.9141, 37.1829)
  line L3586 (-29.9141, 37.1829) -> (-29.7393, 36.9047)
  line L3587 (-29.7393, 36.9047) -> (-29.5344, 36.6479)
  line L3588 (-29.5344, 36.6479) -> (-29.3021, 36.4156)
  line L3589 (-29.3021, 36.4156) -> (-29.0453, 36.2107)
  line L3590 (-29.0453, 36.2107) -> (-28.7671, 36.0359)
  line L3591 (-28.7671, 36.0359) -> (-28.4711, 35.8934)
  line L3592 (-28.4711, 35.8934) -> (-28.161, 35.7849)
  line L3593 (-28.161, 35.7849) -> (-27.8407, 35.7118)
  line L3594 (-27.8407, 35.7118) -> (-27.5143, 35.675)
  line L3595 (-27.5143, 35.675) -> (-27.1857, 35.675)
  line L3596 (-27.1857, 35.675) -> (-26.8593, 35.7118)
  line L3597 (-26.8593, 35.7118) -> (-26.539, 35.7849)
  line L3598 (-26.539, 35.7849) -> (-26.2289, 35.8934)
  line L3599 (-26.2289, 35.8934) -> (-25.9329, 36.0359)
  line L3600 (-25.9329, 36.0359) -> (-25.6547, 36.2107)
  line L3601 (-25.6547, 36.2107) -> (-25.3979, 36.4156)
  line L3602 (-25.3979, 36.4156) -> (-25.1656, 36.6479)
  line L3603 (-25.1656, 36.6479) -> (-24.9607, 36.9047)
  line L3604 (-24.9607, 36.9047) -> (-24.7859, 37.1829)
  line L3605 (-24.7859, 37.1829) -> (-24.6434, 37.4789)
  line L3606 (-24.6434, 37.4789) -> (-24.5349, 37.789)
  line L3607 (-24.5349, 37.789) -> (-24.4618, 38.1093)
  line L3608 (-24.4618, 38.1093) -> (-24.425, 38.4357)
  line L3609 (-24.425, 38.4357) -> (-24.425, 38.7643)
  line L3610 (-24.425, 38.7643) -> (-24.4618, 39.0907)
  line L3611 (-24.4618, 39.0907) -> (-24.5349, 39.411)
  line L3612 (-24.5349, 39.411) -> (-24.5643, 39.495)
  line L3613 (-24.5643, 39.495) -> (-25.3721, 39.495)
  line L3614 (-25.3721, 39.495) -> (-25.3361, 39.4191)
  line L3615 (-25.3361, 39.4191) -> (-25.2495, 39.1512)
  line L3616 (-25.2495, 39.1512) -> (-25.1983, 38.8743)
  line L3617 (-25.1983, 38.8743) -> (-25.1835, 38.5932)
  line L3618 (-25.1835, 38.5932) -> (-25.2053, 38.3125)
  line L3619 (-25.2053, 38.3125) -> (-25.2633, 38.0369)
  line L3620 (-25.2633, 38.0369) -> (-25.3565, 37.7713)
  line L3621 (-25.3565, 37.7713) -> (-25.4834, 37.5199)
  line L3622 (-25.4834, 37.5199) -> (-25.6418, 37.2872)
  line L3623 (-25.6418, 37.2872) -> (-25.829, 37.0769)
  line L3624 (-25.829, 37.0769) -> (-26.042, 36.8927)
  line L3625 (-26.042, 36.8927) -> (-26.277, 36.7377)
  line L3626 (-26.277, 36.7377) -> (-26.5301, 36.6144)
  line L3627 (-26.5301, 36.6144) -> (-26.7971, 36.5251)
  line L3628 (-26.7971, 36.5251) -> (-27.0734, 36.4711)
  line L3629 (-27.0734, 36.4711) -> (-27.3544, 36.4533)
  line L3630 (-27.3544, 36.4533) -> (-27.6353, 36.4722)
  line L3631 (-27.6353, 36.4722) -> (-27.9114, 36.5273)
  line L3632 (-27.9114, 36.5273) -> (-28.1781, 36.6178)
  line L3633 (-28.1781, 36.6178) -> (-28.4307, 36.7421)
  line L3634 (-28.4307, 36.7421) -> (-28.6651, 36.8981)
  line L3635 (-28.6651, 36.8981) -> (-28.8773, 37.0832)
  line L3636 (-28.8773, 37.0832) -> (-29.0637, 37.2942)
  line L3637 (-29.0637, 37.2942) -> (-29.2211, 37.5276)
  line L3638 (-29.2211, 37.5276) -> (-29.347, 37.7794)
  line L3639 (-29.347, 37.7794) -> (-29.4391, 38.0455)
  line L3640 (-29.4391, 38.0455) -> (-29.496, 38.3212)
  line L3641 (-29.496, 38.3212) -> (-29.5166, 38.602)
  line L3642 (-29.5166, 38.602) -> (-29.5006, 38.8831)
  line L3643 (-29.5006, 38.8831) -> (-29.4484, 39.1598)
  line L3644 (-29.4484, 39.1598) -> (-29.3606, 39.4273)
  line L3645 (-29.3606, 39.4273) -> (-29.3282, 39.495)
  line L3646 (-29.3282, 39.495) -> (-30.1357, 39.495)
  line L3647 (-30.1357, 39.495) -> (-30.1651, 39.411)
  line L3648 (-30.1651, 39.411) -> (-30.2382, 39.0907)
  line L3649 (-30.2382, 39.0907) -> (-30.275, 38.7643)
  line L3650 (-30.275, 38.7643) -> (-30.275, 38.4357)
  line L3651 (-26.8401, 42.0374) -> (-26.5056, 41.9709)
  line L3652 (-26.5056, 41.9709) -> (-26.1793, 41.8719)